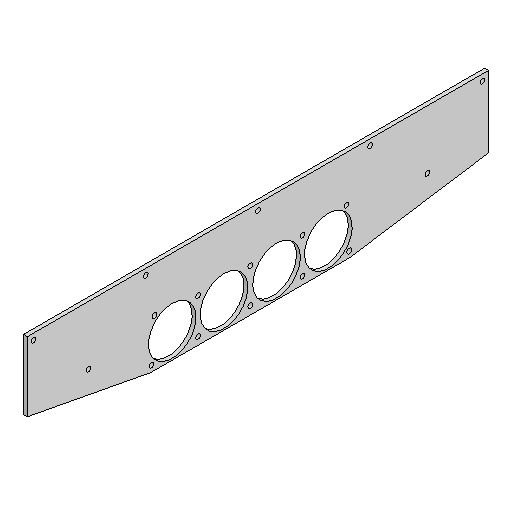
# Autodesk Inventor part: ChassiInsidePlate3.3
Saved by Autodesk Inventor 2023 (Build 270158000, 158)
## iProperties
Created: 2022-11-07
Part Number: ChassiInsidePlate3.3
Material: Generic
Document SubType Name: Modeling
Designer: deli
Density: 1 g/cm^3
Appearance: Default
Author: deli
Autodesk Inventor part; units mm, degrees
ref_plane "YZ Plane" through (0, 0, 0) normal (1, 0, 0) x (0, 1, 0)
ref_plane "XZ Plane" through (0, 0, 0) normal (0, 1, 0) x (-1, 0, 0)
ref_plane "XY Plane" through (0, 0, 0) normal (0, 0, 1) x (1, 0, 0)
sketch "Sketch1" plane through (0, 0, 0) normal (1, 0, 0) x (0, 1, 0)
  arc A0 (527.2714, -141.831) -> (526.2228, -139.2041) centre (525.4336, -141.0418) ccw projected
  arc A1 (218.0959, -5.5727) -> (219.3067, -7.4104) centre (220.0959, -5.5727) ccw projected
  line L0 (218.0959, -5.5727) -> (218.0959, 222.4346) projected
  line L1 (218.0959, 222.4346) -> (133.2497, 222.4346) projected
  line L2 (133.2497, 222.4346) -> (114.1833, 121.8109) projected
  arc A2 (114.1833, 121.8109) -> (114.0959, 120.88) centre (119.0959, 120.88) ccw projected
  arc A3 (114.0959, -41.1964) -> (114.1539, -41.9559) centre (119.0959, -41.1964) ccw projected
  line L3 (114.1539, -41.9559) -> (131.5694, -155.2654) projected
  line L4 (131.5694, -155.2654) -> (216.4156, -155.2654) projected
  circle A4 centre (185.0959, -150.2654) radius 2 projected
  circle A5 centre (185.0959, 125.5096) radius 2 projected
  circle A6 centre (153.0149, 118.2842) radius 2 projected
  circle A7 centre (152.8047, -38.86) radius 2 projected
  circle A8 centre (142.0959, 172.4346) radius 2 projected
  circle A9 centre (142.0959, -105.2654) radius 2 projected
  circle A10 centre (134.8459, 103.7774) radius 4 projected
  circle A11 centre (134.8459, -24.0937) radius 4 projected
  circle A12 centre (149.4359, -2.876) radius 2 projected
  circle A13 centre (120.2559, -2.876) radius 2 projected
  circle A14 centre (185.0959, 217.4346) radius 2 projected
  circle A15 centre (185.0959, -58.3404) radius 2 projected
  circle A16 centre (185.0959, 33.5846) radius 2 projected
  circle A17 centre (119.0959, 120.88) radius 2 projected
  circle A18 centre (119.0959, -41.1964) radius 2 projected
  line L5 (190.0959, 222.4346) -> (190.0959, -155.2654)
  circle A19 centre (134.8459, 103.7774) radius 19.5
  circle A20 centre (134.8459, -24.0937) radius 19.5
  line L6 (526.2228, -139.2041) -> (507.6273, -131.219) projected
  line L7 (114.0959, 120.88) -> (114.0959, -41.1964) projected
  line L8 (216.4156, -155.2654) -> (525.2985, -146.4253) projected
  line L9 (525.2985, -146.4253) -> (527.2714, -141.831) projected
  circle A21 centre (257.9115, -27.7969) radius 1 projected
  circle A22 centre (340.6094, -63.3084) radius 1 projected
  circle A23 centre (437.0902, -104.7385) radius 1 projected
  circle A24 centre (519.788, -140.25) radius 1 projected
  arc A25 (505.1303, -124.9637) -> (507.6273, -131.219) centre (509.5064, -126.8429) ccw projected
  line L10 (505.1303, -124.9637) -> (507.7005, -118.9783) projected
  arc A26 (507.7005, -118.9783) -> (502.1873, -116.6109) centre (504.9439, -117.7946) ccw projected
  line L11 (502.1873, -116.6109) -> (499.6171, -122.5963) projected
  arc A27 (493.3619, -125.0932) -> (499.6171, -122.5963) centre (495.241, -120.7171) ccw projected
  line L12 (493.3619, -125.0932) -> (219.3067, -7.4104) projected
  circle A28 centre (504.9439, -117.7946) radius 1.5 projected
  circle A29 centre (200.5959, 170.2346) radius 1.6 projected
  circle A30 centre (215.5959, 160.2346) radius 1.6 projected
  circle A31 centre (215.5959, 189.1346) radius 1.6 projected
  circle A32 centre (200.5959, 199.1346) radius 1.6 projected
  circle A33 centre (215.5959, 199.1346) radius 1.6 projected
  circle A34 centre (200.5959, 189.1346) radius 1.6 projected
  circle A35 centre (215.5959, 170.2346) radius 1.6 projected
  circle A36 centre (200.5959, 160.2346) radius 1.6 projected
  circle A37 centre (120.2559, 82.5596) radius 2 projected
  circle A38 centre (120.675, 39.8418) radius 2 projected
  circle A39 centre (134.8459, 18.3418) radius 4 projected
  circle A40 centre (134.8459, 61.3418) radius 4 projected
  circle A41 centre (149.0167, 39.8418) radius 2 projected
  circle A42 centre (149.4359, 82.5596) radius 2 projected
  circle A43 centre (134.8459, 61.3418) radius 19.5
  circle A44 centre (134.8459, 18.3418) radius 19.5
  point P0 (0, 0)
  point P1 (114.0959, 111.4062)
  dimension "d0" = 5
  dimension "d1" = 39
  constraints: 4 centre point, 4 coincident, 3 equal radius, 2 end point, 2 point on line, 1 vertical
  measures "d0" distance from line of L5 A5.centre
  measures "d1" diameter of A19
extrude "Extrusion1" add sketch "Sketch1" along normal blind 3.175 contours L4 L3 A3 L7 A2 L2 L1 L5
body "Solid1"
